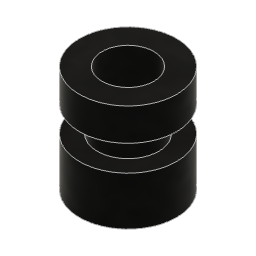
Alu_Endgame (Autodesk Fusion 360 archive; units mm, degrees)
design "M3x6.6 Damper"
Autodesk Fusion 360 part; units mm, degrees
sketch "Sketch1" plane through (0, 0, 0) normal (0, 0, 1) x (1, 0, 0)
  line L0 (0, 3.3) -> (0, -3.3)
  line L1 (0, 3.3) -> (3, 3.3)
  line L2 (3, 3.3) -> (3, 1.3)
  line L3 (3, 1.3) -> (1.9, 1.3)
  line L4 (1.9, 1.3) -> (1.9, -0.3)
  line L5 (1.9, -0.3) -> (3, -0.3)
  line L6 (3, -0.3) -> (3, -3.3)
  line L7 (0, -3.3) -> (3, -3.3)
  dimension "d2" = 6.6
  dimension "d3" = 3.3
  dimension "d4" = 3
  dimension "d5" = 3
  dimension "d6" = 1.6
  dimension "d7" = 1.9
  constraint vertical L0
  constraint perpendicular L0 L1
  constraint perpendicular L1 L2
  constraint perpendicular L2 L3
  constraint perpendicular L3 L4
  constraint perpendicular L4 L5
  constraint perpendicular L3 L6
  constraint perpendicular L6 L7
  constraint coincident origin L0
  constraint equal L1 L7
  measures "d2" distance of L0.start L0.end
  measures "d3" distance of origin L0.start
  measures "d4" distance of L0.start L1.end
  measures "d5" distance of L5.end L6.end
  measures "d6" distance of L3.end L4.end
  measures "d7" distance of L0 L4
revolve "Revolve1" add sketch "Sketch1" angle 360 about axis through (0, 3.3, 0) along (0, -1, 0)
sketch "Sketch2" plane through (0, 3.3, 0) normal (0, 1, 0) x (-1, 0, 0)
  circle A0 centre (0, 0) radius 3
  circle A1 centre (0, 0) radius 1.6
  dimension "d9" = 3.2
  constraint coincident A0.centre A1.centre
  measures "d9" diameter of A1
extrude "Extrude1" cut sketch "Sketch2" against normal through all contours A1
equation "d3 = d2 / 2"
equation "d7 = ( 3.8 / 2 ) * 1 mm"
